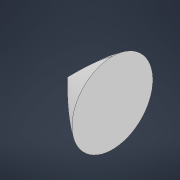
# Autodesk Inventor part: sincos half
Saved by Autodesk Inventor 2022 (Build 260153000, 153)
## iProperties
Created: 2021-06-07
Part Number: sincos half
Material: Generic
Document SubType Name: Modeling
Designer: sidsa
Density: 1 g/cm^3
Appearance: Default
Author: sidsa
## iProperties of the stored document sincos half_3DPrint.ipt
Created: 2021-06-07
Part Number: sincos half_3DPrint
Material: Generic
Document SubType Name: Modeling
Designer: sidsa
Density: 1 g/cm^3
Appearance: Default
Author: sidsa
Autodesk Inventor part; units mm, degrees
ref_plane "YZ Plane" through (0, 0, 0) normal (1, 0, 0) x (0, 1, 0)
ref_plane "XZ Plane" through (0, 0, 0) normal (0, 1, 0) x (-1, 0, 0)
ref_plane "XY Plane" through (0, 0, 0) normal (0, 0, 1) x (1, 0, 0)
sketch "Sketch1" plane through (0, 0, 0) normal (0, 0, 1) x (1, 0, 0)
  spline S0 degree 5 poles (0, 0) (2.6013, 2.6012) (5.2018, 5.2026) (7.8323, 7.7749) (12.8937, 12.5179) (18.2925, 16.8751) (20.922, 18.7976) (26.0439, 22.0276) (31.6582, 24.2654) (34.3546, 25.022) (39.897, 25.778) (45.4395, 25.022) (48.1359, 24.2654) (53.7502, 22.0276) (58.8721, 18.7976) (61.5016, 16.8751) (66.9004, 12.5179) (71.9618, 7.7749) (74.5923, 5.2026) (77.1928, 2.6012) (79.7941, 0) knots 0 0 0 0 0 0 0.189558 0.189558 0.189558 0.35722 0.35722 0.35722 0.5 0.5 0.5 0.64278 0.64278 0.64278 0.810442 0.810442 0.810442 1 1 1 1 1 1
  spline S1 degree 5 poles (0, 25.4) (2.7702, 25.4001) (5.5445, 25.0219) (8.2382, 24.2654) (13.8544, 22.0273) (18.9751, 18.7972) (21.6054, 16.8746) (27.0038, 12.5172) (32.0659, 7.774) (34.6961, 5.2016) (37.2969, 2.6001) (39.8982, -0.0012) knots 0 0 0 0 0 0 0.285559 0.285559 0.285559 0.620883 0.620883 0.620883 1 1 1 1 1 1
  line L0 (0, 0) -> (39.8982, 0)
  line L1 (19.9487, 17.9606) -> (19.9491, 0)
  point P0 (19.9487, 17.9606)
  constraints: 4 end point, 1 horizontal, 1 midpoint, 8 other
revolve "Revolution2" add sketch "Sketch1" angle 360 about axis through (0, 0, 0) along (1, 0, 0) contours S0 L1 L0
equation "curve S0 of \"Sketch1\": x = t; y = 1 in * sin(t * 180 / 3.1415); t from d0 to d1"
equation "curve S1 of \"Sketch1\": x = t; y = cos(t * 180 / 3.1415); t from d2 to d3"
body "Solid2"
